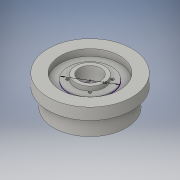
# Autodesk Inventor part: Part1
Saved by Autodesk Inventor 2016 (Build 200138000, 138)
## iProperties
Created: 2018-01-17
Part Number: Part1
Material: Generic
Document SubType Name: Modeling
Designer: John
Density: 1 g/cm^3
Appearance: Default
Author: John
Autodesk Inventor part; units mm, degrees
ref_plane "YZ Plane" through (0, 0, 0) normal (1, 0, 0) x (0, 1, 0)
ref_plane "XZ Plane" through (0, 0, 0) normal (0, 1, 0) x (-1, 0, 0)
ref_plane "XY Plane" through (0, 0, 0) normal (0, 0, 1) x (1, 0, 0)
sketch "Sketch1" plane through (0, 0, 0) normal (0, 1, 0) x (-1, 0, 0)
  circle A0 centre (0, 0) radius 58
  dimension "d0" = 116
  constraints: 1 centre point, 1 coincident
  measures "d0" diameter of A0
extrude "Extrusion1" add sketch "Sketch1" along normal blind 16
sketch "Sketch2" plane through (0, 16, 0) normal (0, 1, 0) x (1, 0, 0)
  circle A0 centre (0, 0) radius 41
  dimension "d3" = 82
  constraints: 1 centre point, 1 coincident
  measures "d3" diameter of A0
extrude "Extrusion2" cut sketch "Sketch2" against normal blind 9
sketch "Sketch3" plane through (0, 0, 0) normal (0, -1, 0) x (1, 0, 0)
  circle A0 centre (0, 0) radius 50
  dimension "d6" = 100
  constraints: 1 centre point, 1 coincident
  measures "d6" diameter of A0
extrude "Extrusion3" add sketch "Sketch3" along normal blind 25
sketch "Sketch4" plane through (0, 7, 0) normal (0, 1, 0) x (1, 0, 0)
  circle A0 centre (0, 0) radius 30
  dimension "d9" = 60
  constraints: 1 centre point, 1 coincident
  measures "d9" diameter of A0
extrude "Extrusion4" add sketch "Sketch4" along normal blind 1.3
sketch "Sketch6" plane through (0, 8.3, 0) normal (0, 1, 0) x (1, 0, 0)
  circle A0 centre (0, 0) radius 20
  dimension "d12" = 40
  constraints: 1 centre point, 1 coincident
  measures "d12" diameter of A0
extrude "Extrusion5" add sketch "Sketch6" along normal blind 6
sketch "Sketch7" plane through (0, 14.3, 0) normal (0, 1, 0) x (1, 0, 0)
  circle A0 centre (0, 0) radius 15
  dimension "d15" = 30
  constraints: 1 centre point, 1 coincident
  measures "d15" diameter of A0
extrude "Extrusion6" cut sketch "Sketch7" against normal blind 50
sketch "Sketch8" plane through (0, -25, 0) normal (0, -1, 0) x (1, 0, 0)
  line L0 (-22, 22) -> (22, 22)
  line L1 (22, 22) -> (22, -22)
  line L2 (22, -22) -> (-22, -22)
  line L3 (-22, -22) -> (-22, 22)
  circle A0 centre (0, 0) radius 20 projected
  point P0 (-15.5, 15.5)
  point P1 (15.5, 15.5)
  point P2 (15.5, -15.5)
  point P3 (-15.5, -15.3905)
  dimension "d34" = 22
  dimension "d35" = 22
  dimension "d36" = 22
  dimension "d37" = 22
  constraints: 8 end point, 2 parallel, 1 horizontal, 1 perpendicular
  measures "d34" distance from line of point (0, 0) L3
  measures "d35" distance from line of point (0, 0) L1
  measures "d36" distance from line of point (0, 0) L2
  measures "d37" distance from line of point (0, 0) L0
extrude "Extrusion7" cut sketch "Sketch8" against normal blind 20 contours L0 L1 L2 L3 | A0
sketch "Sketch12" plane through (0, 8.3, 0) normal (0, 1, 0) x (1, 0, 0)
  point P0 (0, 0)
  point P1 (-15.5, 15.5)
  point P2 (15.5, 15.5)
  point P3 (15.5, -15.5)
  point P4 (-15.5, -15.5)
  dimension "d72" = 31
  dimension "d73" = 31
  dimension "d74" = 31
  dimension "d75" = 31
  dimension "d76" = 15.5
  dimension "d77" = 15.5
  dimension "d85" = 15.5
  measures "d72" distance of point (15.5, 15.5) point (-15.5, 15.5)
  measures "d73" distance of point (15.5, -15.5) point (15.5, 15.5)
  measures "d74" distance of point (-15.5, -15.5) point (15.5, -15.5)
  measures "d75" distance of point (-15.5, 15.5) point (-15.5, -15.5)
  measures "d76" horizontal distance of point (0, 0) point (-15.5, 15.5)
  measures "d77" horizontal distance of point (0, 0) point (-15.5, 15.5)
  measures "d85" horizontal distance of point (0, 0) point (-15.5, -15.5)
hole "Hole5" at (-15.5, 8.3, -15.5) at (15.5, 8.3, -15.5) at (15.5, 8.3, 15.5) at (-15.5, 8.3, 15.5) direction (0, -1, 0) diameter 3 end through all counterbore diameter 4 counterbore depth 2
body "Solid1"
